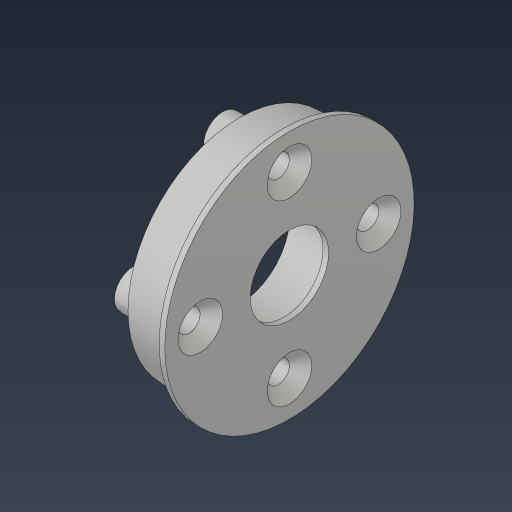
# Autodesk Inventor part: Getriebe Abdeckung
Saved by Autodesk Inventor 2023.1 (Build 271208000, 208)
## iProperties
Part Number: Getriebe Abdeckung
Material: Aluminium 6061
Document SubType Name: Modeling
Designer: rYan
Mass: 3.49086 g
Surface Area: 10.6125 cm^2
Volume: 1.29291 cm^3
Density: 2.7 g/cm^3
Appearance: Aluminium - flach
Author: rYan
Autodesk Inventor part; units mm, degrees
ref_plane "YZ Plane" through (0, 0, 0) normal (1, 0, 0) x (0, 1, 0)
ref_plane "XZ Plane" through (0, 0, 0) normal (0, 1, 0) x (-1, 0, 0)
ref_plane "XY Plane" through (0, 0, 0) normal (0, 0, 1) x (1, 0, 0)
sketch "Skizze1" plane through (0, 0, 0) normal (0, 1, 0) x (-1, 0, 0)
  line L0 (0, 11.18) -> (0.5, 11.18)
  line L1 (0.5, 11.18) -> (0.5, 9.98)
  line L2 (0.5, 9.98) -> (4.5, 9.98)
  line L3 (4.5, 9.98) -> (4.5, 4.515)
  line L4 (4.5, 4.515) -> (0.5, 4.515)
  line L5 (0.5, 4.515) -> (0.5, 3.515)
  line L6 (0.5, 3.515) -> (0, 3.515)
  line L7 (0, 3.515) -> (0, 11.18)
  line L8 (0, 0) -> (7.49, 0)
  dimension "d1" = 9.03
  dimension "d2" = 1
  dimension "d3" = 4
  dimension "d5" = 19.96
  dimension "d6" = 1.2
  dimension "d7" = 4
  dimension "d9" = 0.5
  constraints: 18 end point, 6 perpendicular, 1 horizontal, 1 point on line
  measures "d1" diameter of L4 L8
  measures "d2" distance between parallel lines of L6 L4
  measures "d3" distance of L3.end L4.end
  measures "d5" diameter of L2 L8
  measures "d6" distance between parallel lines of L0 L2
  measures "d7" distance of L1.end L2.end
  measures "d9" distance between parallel lines of L7 L1
revolve "Umdrehung1" add sketch "Skizze1" angle 360 about axis through (0, 0, 0) along (-1, 0, 0)
sketch "Skizze2" plane through (0, 0, 0) normal (1, 0, 0) x (0, 0, -1)
  line L0 (-15.652, 0) -> (15.652, 0) projected
  point P0 (0, 0)
  point P1 (-8, 0)
  dimension "d11" = 8
  constraints: 1 point on line
  measures "d11" distance of point (0, 0) point (-8, 0)
hole "Bohrung1" at (0, 0, 8) direction (-1, 0, 0) diameter 2 depth 5 tip angle 118 countersink diameter 4 countersink angle 90
sketch "Skizze4" plane through (-4.5, 0, 0) normal (-1, 0, 0) x (0, 0, 1)
  circle A0 centre (8, 0) radius 1 projected
  circle A1 centre (8, 0) radius 1.7
  point P0 (0, 0)
  dimension "d22" = 3.4
  constraints: 1 centre point, 1 coincident
  measures "d22" diameter of A1
extrude "Extrusion1" add sketch "Skizze4" along normal blind 1.5
pattern_circular "Runde Anordnung1" count 4 over 360 about axis through (-10, 0, 0) along (1, 0, 0) of "Bohrung1", "Extrusion1"
